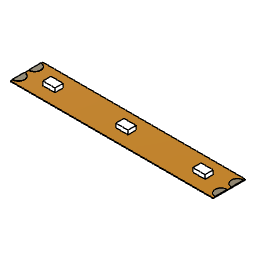
5_segment_IP20_60_LEDs_per_m_12V_cool_white_LED_strip (Autodesk Fusion 360 archive; units mm, degrees)
design "LED Strip"
Autodesk Fusion 360 part; units mm, degrees
sketch "strip" plane through (0, 0, 0) normal (0, 0, 1) x (1, 0, 0)
  line L0 (0, 0) -> (50, 0)
  line L1 (50, 0) -> (50, 8)
  line L2 (50, 8) -> (0, 8)
  line L3 (0, 8) -> (0, 0)
  dimension "d1" = 50
  dimension "d2" = 8
  constraint horizontal L0
  constraint vertical L1
  constraint horizontal L2
  constraint vertical L3
  constraint coincident L0.start L3.end
  measures "d1" distance of L0.start L0.end
  measures "d2" distance of L0.end L1.end
extrude "Extrude1" add sketch "strip" along normal blind 0.1 makes body 1
sketch "leds" plane through (0, 0, 0.1) normal (0, 0, 1) x (-1, 0, 0)
  line L0 (0, -8) -> (0, 0)
  line L1 (0, 0) -> (-50, 0)
  line L2 (-50, 0) -> (-50, -8)
  line L3 (-50, -8) -> (0, -8)
  line L4 (-5, -5) -> (-8, -5)
  line L5 (-8, -5) -> (-8, -3)
  line L6 (-8, -3) -> (-5, -3)
  line L7 (-5, -3) -> (-5, -5)
  line L8 (-23, -5) -> (-26, -5)
  line L9 (-26, -5) -> (-26, -3)
  line L10 (-26, -3) -> (-23, -3)
  line L11 (-23, -3) -> (-23, -5)
  line L12 (-42, -5) -> (-45, -5)
  line L13 (-45, -5) -> (-45, -3)
  line L14 (-45, -3) -> (-42, -3)
  line L15 (-42, -3) -> (-42, -5)
  dimension "d6" = 5
  dimension "d7" = 15
  dimension "d8" = 3
  dimension "d9" = 3
  dimension "d10" = 3
  dimension "d11" = 5
  dimension "d12" = 16
  dimension "d13" = 2
  dimension "d14" = 2
  dimension "d15" = 2
  dimension "d16" = 3
  constraint horizontal L4
  constraint vertical L5
  constraint horizontal L6
  constraint vertical L7
  constraint horizontal L8
  constraint vertical L9
  constraint horizontal L10
  constraint vertical L11
  constraint horizontal L12
  constraint vertical L13
  constraint horizontal L14
  constraint vertical L15
  constraint collinear L4 L8
  measures "d6" distance of L0 L7
  measures "d7" distance of L5 L11
  measures "d8" distance of L5.end L6.end
  measures "d9" distance of L9.end L10.end
  measures "d10" distance of L13.end L14.end
  measures "d11" distance of L2 L13
  measures "d12" distance of L9 L15
  measures "d13" distance of L4.start L6.end
  measures "d14" distance of L8.start L10.end
  measures "d15" distance of L12.start L14.end
  measures "d16" distance of L3 L4
extrude "Extrude2" add sketch "leds" along normal blind 1 separate body contours L4 L5 L6 L7 | L8 L9 L10 L11 | L12 L13 L14 L15 makes body 2 at (6, 4.3333, 0.1) makes body 3 at (24, 4.3333, 0.1) makes body 4 at (43, 4.3333, 0.1)
sketch "Sketch3" plane through (0, 0, 0.1) normal (0, 0, 1) x (-1, 0, 0)
  line L0 (0, -8) -> (0, 0)
  line L1 (0, 0) -> (-50, 0)
  line L2 (-50, 0) -> (-50, -8)
  line L3 (-50, -8) -> (0, -8)
  circle A0 centre (0, -6) radius 1.5
  circle A1 centre (0, -2) radius 1.5
  circle A2 centre (-50, -6) radius 1.5
  circle A3 centre (-50, -2) radius 1.5
  dimension "d19" = 3
  dimension "d20" = 3
  dimension "d21" = 3
  dimension "d22" = 3
  dimension "d23" = 2
  dimension "d24" = 2
  dimension "d25" = 2
  dimension "d26" = 2
  constraint coincident L2 A2.centre
  constraint coincident L2 A3.centre
  measures "d19" diameter of A2
  measures "d20" diameter of A3
  measures "d21" diameter of A0
  measures "d22" diameter of A1
  measures "d23" distance of L3 A2.centre
  measures "d24" distance of L1 A3.centre
  measures "d25" distance of L3 A0.centre
  measures "d26" distance of L1 A1.centre
extrude "Extrude3" add sketch "Sketch3" along normal blind 0.1 separate body contours L0 A0 | L2 A2 | L0 A1 | L2 A3 picked at (-0.4654, -6.1827) picked at (-49.0815, -5.6726) picked at (-0.2169, -2.4505) picked at (-49.0815, -1.6726) makes body 5 at (0.4654, 6.1827, 0.1) makes body 6 at (49.1724, 2.4778, 0.2) makes body 7 at (0.2169, 2.4505, 0.1) makes body 8 at (49.2956, 5.6062, 0.1)
named bodies: "strip", "left led", "middle led", "right led", "connector top left", "connector bottom right", "connector bottom left", "connector top right"
